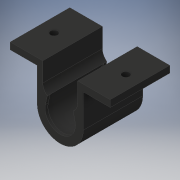
# Autodesk Inventor part: Heated Bed Bearing Mount
Saved by Autodesk Inventor 2019.4 (Build 234330000, 330)
## iProperties
Created: 2018-08-19
Part Number: Heated Bed Bearing Mount
Material: Generic
Document SubType Name: Modeling
Designer: Richard
Density: 1 g/cm^3
Appearance: Rubber - Black
Author: Richard
Autodesk Inventor part; units mm, degrees
ref_plane "YZ Plane" through (0, 0, 0) normal (1, 0, 0) x (0, 1, 0)
ref_plane "XZ Plane" through (0, 0, 0) normal (0, 1, 0) x (-1, 0, 0)
ref_plane "XY Plane" through (0, 0, 0) normal (0, 0, 1) x (1, 0, 0)
sketch "Sketch1" plane through (0, 0, 0) normal (0, 0, 1) x (1, 0, 0)
  line L0 (-22.25, 17.75) -> (-22.25, 14.75)
  line L1 (-22.25, 14.75) -> (-10.25, 14.75)
  line L2 (-10.25, 14.75) -> (-10.25, 0)
  arc A0 (-10.25, 0) -> (10.25, 0) centre (0, 0) ccw
  line L3 (10.25, 0) -> (10.25, 14.75)
  line L4 (10.25, 14.75) -> (22.25, 14.75)
  line L5 (22.25, 14.75) -> (22.25, 17.75)
  line L6 (22.25, 17.75) -> (-22.25, 17.75)
  point P0 (0, 17.75)
  dimension "d0" = 44.5
  dimension "d1" = 10.25
  dimension "d2" = 3
  dimension "d3" = 17.75
  constraints: 14 end point, 4 perpendicular, 2 point on circle, 2 point on line, 2 tangent, 1 centre point, 1 coincident, 1 midpoint, 1 parallel, 1 vertical, 1 vertical alignment
  measures "d0" distance of L5.end L0.start
  measures "d1" radius of A0
  measures "d2" distance of L0.start L0.end
  measures "d3" distance from line of point (0, 0) L6
extrude "Extrusion1" add sketch "Sketch1" along normal mid plane 26.5
sketch "Sketch2" plane through (0, 0, 13.25) normal (0, 0, 1) x (1, 0, 0)
  line L0 (-22.25, 17.75) -> (-22.25, 14.75) construction
  line L1 (-22.25, 14.75) -> (-10.25, 14.75) construction
  line L2 (-10.25, 14.75) -> (-10.25, 0) construction
  arc A0 (-10.25, 0) -> (10.25, 0) centre (0, 0) ccw construction
  line L3 (10.25, 0) -> (10.25, 14.75) construction
  line L4 (10.25, 14.75) -> (22.25, 14.75) construction
  line L5 (22.25, 14.75) -> (22.25, 17.75) construction
  line L6 (22.25, 17.75) -> (-22.25, 17.75) construction
  line L7 (-7.75, 17.75) -> (7.75, 17.75)
  line L8 (7.75, 17.75) -> (7.75, 9.1962)
  arc A1 (5.75, 5.1962) -> (7.75, 9.1962) centre (2.75, 9.1962) ccw
  line L9 (5.75, 5.1962) -> (6.5855, 1.4811)
  arc A2 (-6.5855, 1.4811) -> (6.5855, 1.4811) centre (0, 0) ccw
  line L10 (-6.5855, 1.4811) -> (-5.75, 5.1962)
  arc A3 (-7.75, 9.1962) -> (-5.75, 5.1962) centre (-2.75, 9.1962) ccw
  line L11 (-7.75, 9.1962) -> (-7.75, 17.75)
  line L12 (22.25, 17.75) -> (-22.25, 17.75) projected
  point P0 (0, 17.75)
  dimension "d6" = 5
  dimension "d7" = 6.75
  dimension "d8" = 2.5
  dimension "d9" = 11.5
  dimension "d10" = 7.75
  constraints: 10 end point, 6 point on circle, 4 tangent, 3 centre point, 2 equal length, 1 coincident, 1 collinear, 1 equal radius, 1 horizontal, 1 horizontal alignment, 1 midpoint, 1 perpendicular, 1 vertical, 1 vertical alignment
  measures "d6" radius of A3
  measures "d7" radius of A2
  measures "d8" distance between parallel lines of L2 L11
  measures "d9" distance of L9.start L10.end
  measures "d10" distance of point (0, 0) L10.end
extrude "Extrusion2" cut sketch "Sketch2" against normal blind 26.5
sketch "Sketch3" plane through (0, 0, 0) normal (0, 0, 1) x (1, 0, 0)
  circle A0 centre (0, 0) radius 7.75
  dimension "d13" = 15.5
  constraints: 1 centre point, 1 coincident
  measures "d13" diameter of A0
extrude "Extrusion3" cut sketch "Sketch3" along normal mid plane 24
sketch "Sketch4" plane through (-22.25, 17.75, 13.25) normal (0, 1, 0) x (1, 0, 0)
  line L0 (0, 26.5) -> (14.5, 26.5) projected
  line L1 (44.5, 26.5) -> (44.5, 0) projected
  point P0 (22.25, 13.25)
  point P1 (0, 0)
  point P2 (6.25, 13.25)
  point P3 (38.25, 13.25)
  dimension "d16" = 6.25
  dimension "d17" = 13.25
  dimension "d19" = 6.25
  constraints: 1 horizontal alignment
  measures "d16" horizontal distance of point (0, 0) point (6.25, 13.25)
  measures "d17" vertical distance of point (0, 0) point (6.25, 13.25)
  measures "d19" distance from line of L1 point (38.25, 13.25)
hole "Hole1" at (-16, 17.75, 0) at (16, 17.75, 0) direction (0, -1, 0) diameter 3.2 end through all
equation "\"d19\" = d16"
body "Solid1"
